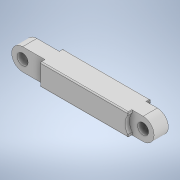
# Autodesk Inventor part: New_ThinArm_first
Saved by Autodesk Inventor 2021 (Build 250183000, 183)
## iProperties
Created: 2021-08-05
Part Number: New_ThinArm_first
Material: Generic
Document SubType Name: Modeling
Designer: hp
Density: 1 g/cm^3
Appearance: Default
Author: hp
Autodesk Inventor part; units mm, degrees
ref_plane "YZ Plane" through (0, 0, 0) normal (1, 0, 0) x (0, 1, 0)
ref_plane "XZ Plane" through (0, 0, 0) normal (0, 1, 0) x (-1, 0, 0)
ref_plane "XY Plane" through (0, 0, 0) normal (0, 0, 1) x (1, 0, 0)
sketch "Sketch1" plane through (0, 0, 0) normal (0, 0, 1) x (1, 0, 0)
  circle A0 centre (0, 0) radius 2
  circle A1 centre (0, 0) radius 1
  line L0 (0, 0) -> (22, 0)
  circle A2 centre (22, 0) radius 1
  circle A3 centre (22, 0) radius 2
  line L1 (0, 2) -> (22, 2)
  line L2 (0, -2) -> (22, -2)
  dimension "d0" = 4
  dimension "d1" = 2
  dimension "d2" = 22
  dimension "d3" = 2
  dimension "d4" = 4
  constraints: 6 end point, 4 centre point, 4 coincident, 4 point on circle, 2 tangent, 1 horizontal
  measures "d0" diameter of A0
  measures "d1" diameter of A1
  measures "d2" distance of L0.start L0.end
  measures "d3" diameter of A2
  measures "d4" diameter of A3
extrude "Extrusion1" add sketch "Sketch1" along normal mid plane 2.6
sketch "Sketch3" plane through (0, 0, 0) normal (0, 0, 1) x (1, 0, 0)
  line L0 (0, 0) -> (4, 0)
  line L1 (4, 0) -> (4, 2)
  line L2 (22, 2) -> (0, 2) projected
  line L3 (4, 0) -> (4, -2)
  line L4 (0, -2) -> (22, -2) projected
  line L5 (4, 0) -> (20, 0)
  line L6 (20, 0) -> (20, 2)
  line L7 (20, 0) -> (20, -2)
  circle A0 centre (22, 0) radius 2.5
  point P0 (20, 1.5)
  point P1 (20, -1.5)
  dimension "d16" = 4
  dimension "d17" = 5
  constraints: 12 end point, 4 point on line, 2 horizontal, 2 perpendicular, 1 centre point, 1 vertical
  measures "d16" distance of L0.start L0.end
  measures "d17" diameter of A0
extrude "Extrusion3" add sketch "Sketch3" along normal mid plane 4.2 contours L5 A0 L7 L4 L3 | L1 L2 L6 A0 L5
fillet "Fillet3" radius 0.2 4 edges at (12, 2, 2.1) (12, -2, 2.1) (12, -2, -2.1) (12, 2, -2.1)
fillet "Fillet4" radius 0.1 20 edges at (20, 1.9414, 2.0414) (20, 2, 1.6) (20, 1.65, 2.1) (20, -1.65, 2.1) (20, -2, 1.6) (20, -1.9414, 2.0414) (20, 1.65, -2.1) (20, 2, -1.6) (20, 1.9414, -2.0414) (20, -1.9414, -2.0414) (20, -2, -1.6) (20, -1.65, -2.1) (4, 2, -1.6) (4, 0, -2.1) (4, -2, 1.6) (4, -2, -1.6) (4, 1.9414, -2.0414) (4, 1.9414, 2.0414) (4, 0, 2.1) (4, 2, 1.6)
body "Solid1"
